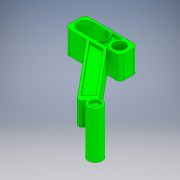
# Autodesk Inventor part: finger_4_6mm
Saved by Autodesk Inventor 2018 (Build 220112000, 112)
## iProperties
Created: 2019-01-24
Part Number: finger_4_6mm
Material: 一般
Document SubType Name: Modeling
Designer: lowyu
Density: 1 g/cm^3
Appearance: 既定
Author: lowyu
## iProperties of the stored document finger_4_6mm_3D プリント.ipt
Created: 2019-01-24
Part Number: finger_4_6mm_3D プリント
Material: 一般
Document SubType Name: Modeling
Designer: lowyu
Density: 1 g/cm^3
Appearance: 既定
Author: lowyu
Autodesk Inventor part; units mm, degrees
ref_plane "YZ Plane" through (0, 0, 0) normal (1, 0, 0) x (0, 1, 0)
ref_plane "XZ Plane" through (0, 0, 0) normal (0, 1, 0) x (-1, 0, 0)
ref_plane "XY Plane" through (0, 0, 0) normal (0, 0, 1) x (1, 0, 0)
sketch "スケッチ1" plane through (0, 0, 0) normal (0, 0, 1) x (1, 0, 0)
  line L0 (18.4549, -7.695) -> (14.2688, -7.695)
  arc A0 (18.4549, -7.695) -> (20.0703, -6.0796) centre (18.4549, -6.0796) ccw
  line L1 (20.0703, -2.0624) -> (20.0703, -6.0796)
  line L2 (18.0495, -0.0417) -> (-1.0589, -0.0417)
  arc A1 (-1.0589, -0.0417) -> (-2.9016, -1.8843) centre (-1.0589, -1.8843) ccw
  line L3 (-2.9016, -1.8843) -> (-2.9016, -6.5999)
  arc A2 (-2.9016, -6.5999) -> (-0.7003, -8.8011) centre (-0.7003, -6.5999) ccw
  arc A3 (26.8872, -33.0759) -> (27.9503, -33.1763) centre (27.7277, -29.8571) ccw
  line L4 (29.6628, -31.7291) -> (27.9503, -33.1763)
  arc A4 (29.6628, -31.7291) -> (31.463, -28.2522) centre (32.5816, -31.0359) ccw
  line L5 (31.463, -28.2522) -> (14.2688, -7.695)
  circle A5 centre (16.1123, -4.0657) radius 2.5
  line L6 (7.6373, -0.9827) -> (1.1644, -0.9827)
  arc A6 (7.6373, -7.2327) -> (7.6373, -0.9827) centre (7.6373, -4.1077) ccw
  arc A7 (1.1644, -0.9827) -> (1.1644, -7.2327) centre (1.1644, -4.1077) ccw
  line L7 (26.8872, -33.0759) -> (6.5837, -8.8011)
  line L8 (-0.7003, -8.8011) -> (6.5837, -8.8011)
  arc A8 (20.0703, -2.0624) -> (18.0495, -0.0417) centre (18.0495, -2.0624) ccw
  line L9 (1.1644, -7.2327) -> (7.6373, -7.2327)
  line L10 (13.6123, -4.0657) -> (13.6123, 1.3375)
  line L11 (10.7623, -4.0657) -> (10.7623, 0.9924)
  point P0 (0, 0)
  point P1 (0, 0)
  point P2 (0, 0)
  dimension "d0" = 5
  dimension "d1" = 3.125
  dimension "d2" = 4.8539
  dimension "d3" = 4.066
  dimension "d4" = 4.066
  dimension "d5" = 90
  dimension "d6" = 90
  dimension "d7" = 3.125
  dimension "d8" = 3.9579
  dimension "d9" = 22.9718
  dimension "d10" = 3
  dimension "d11" = 2.85
  constraints: 24 end point, 16 point on circle, 11 tangent, 8 centre point, 4 parallel, 2 horizontal, 2 perpendicular, 1 coincident, 1 horizontal alignment, 1 vertical, 2 other
  measures "d1" radius of A6
  measures "d2" horizontal distance of A4.centre A3.centre
  measures "d3" distance from line of L2 A7.centre
  measures "d4" distance from line of L3 A7.centre
  measures "d7" radius of A7
  measures "d8" distance from line of L1 point (16.112, -4.066)
  measures "d9" distance between parallel lines of L1 L3
  measures "d10" radius of A4
  measures "d11" distance between parallel lines of L10 L11
extrude "押し出し1" add sketch "スケッチ1" along normal blind 10
sketch "スケッチ2" plane through (0, 0, 0) normal (0, 0, -1) x (-1, 0, 0)
  arc A0 (-31.463, -28.2522) -> (-29.6628, -31.7291) centre (-32.5816, -31.0359) ccw projected
  circle A1 centre (-32.5816, -31.0359) radius 3
  point P0 (0, 0)
  constraints: 1 centre point, 1 coincident, 1 concentric
extrude "押し出し2" add sketch "スケッチ2" along normal blind 10
sketch "スケッチ3" plane through (0, 0, 10) normal (0, 0, 1) x (1, 0, 0)
  line L0 (6.5837, -8.8011) -> (26.8872, -33.0759) projected
  line L1 (31.463, -28.2522) -> (14.2688, -7.695) projected
  line L2 (6.5837, -8.8011) -> (15.194, -8.8011)
  line L3 (26.8872, -33.0759) -> (31.463, -28.2522)
  line L4 (31.463, -28.2522) -> (15.194, -8.8011)
  line L5 (26.8872, -33.0759) -> (6.5837, -8.8011)
  line L6 (25.9184, -31.9176) -> (30.4942, -27.0939)
  line L7 (26.6112, -31.1873) -> (7.8873, -8.8011)
  line L8 (29.8014, -27.8243) -> (13.8903, -8.8011)
  point P0 (0, 0)
  dimension "d16" = 1.5
  dimension "d17" = 1
  dimension "d18" = 1
  constraints: 14 end point, 7 point on line, 3 parallel, 1 collinear, 1 horizontal
  measures "d16" distance between parallel lines of L3 L6
  measures "d17" distance between parallel lines of L0 L7
  measures "d18" distance between parallel lines of L1 L8
extrude "押し出し3" cut sketch "スケッチ3" against normal blind 1 contours L2 L8 L6 L7
sketch "スケッチ4" plane through (0, 0, 10) normal (0, 0, 1) x (1, 0, 0)
  arc A0 (7.6373, -7.2327) -> (7.6373, -0.9827) centre (7.6373, -4.1077) ccw projected
  circle A1 centre (16.1123, -4.0657) radius 2.5 projected
  line L0 (18.0495, -0.0417) -> (-1.0589, -0.0417) projected
  line L1 (14.2688, -7.695) -> (18.4549, -7.695) projected
  line L2 (7.8873, -8.8011) -> (13.8903, -8.8011) projected
  line L3 (13.8903, -8.8011) -> (29.8014, -27.8243) projected
  line L4 (29.8014, -27.8243) -> (26.6112, -31.1873) projected
  line L5 (26.6112, -31.1873) -> (7.8873, -8.8011) projected
  line L6 (7.8873, -8.8011) -> (13.8903, -8.8011) projected
  arc A2 (7.6373, -7.2327) -> (7.6373, -0.9827) centre (7.6373, -4.1077) ccw projected
  line L7 (7.6373, -7.2327) -> (1.1644, -7.2327) projected
  arc A3 (1.1644, -0.9827) -> (1.1644, -7.2327) centre (1.1644, -4.1077) ccw projected
  line L8 (1.1644, -0.9827) -> (7.6373, -0.9827) projected
  circle A4 centre (16.1123, -4.0657) radius 2.5 projected
  line L9 (14.2688, -7.695) -> (18.4549, -7.695) projected
  arc A5 (18.4549, -7.695) -> (20.0703, -6.0796) centre (18.4549, -6.0796) ccw projected
  line L10 (20.0703, -6.0796) -> (20.0703, -2.0624) projected
  arc A6 (20.0703, -2.0624) -> (18.0495, -0.0417) centre (18.0495, -2.0624) ccw projected
  line L11 (18.0495, -0.0417) -> (-1.0589, -0.0417) projected
  arc A7 (-1.0589, -0.0417) -> (-2.9016, -1.8843) centre (-1.0589, -1.8843) ccw projected
  line L12 (-2.9016, -1.8843) -> (-2.9016, -6.5999) projected
  arc A8 (-2.9016, -6.5999) -> (-0.7003, -8.8011) centre (-0.7003, -6.5999) ccw projected
  line L13 (-0.7003, -8.8011) -> (6.5837, -8.8011) projected
  line L14 (6.5837, -8.8011) -> (26.8872, -33.0759) projected
  arc A9 (26.8872, -33.0759) -> (27.9503, -33.1763) centre (27.7277, -29.8571) ccw projected
  line L15 (27.9503, -33.1763) -> (29.6628, -31.7291) projected
  arc A10 (29.6628, -31.7291) -> (31.463, -28.2522) centre (32.5816, -31.0359) ccw projected
  line L16 (31.463, -28.2522) -> (14.2688, -7.695) projected
  arc A11 (9.5454, -7.2327) -> (9.5355, -0.9767) centre (7.6373, -4.1077) ccw
  arc A12 (14.3143, -0.9767) -> (14.4552, -7.2327) centre (16.1123, -4.0657) ccw
  line L17 (9.5454, -7.2327) -> (14.4552, -7.2327)
  line L18 (9.5355, -0.9767) -> (14.3143, -0.9767)
  point P0 (0, 0)
  constraints: 5 point on circle, 4 end point, 2 centre point, 2 coincident, 2 horizontal
extrude "押し出し4" cut sketch "スケッチ4" against normal blind 1 contours A11 L18 A12 L17
sketch "スケッチ5" plane through (0, 0, 10) normal (0, 0, 1) x (1, 0, 0)
  arc A0 (29.6628, -31.7291) -> (31.463, -28.2522) centre (32.5816, -31.0359) ccw projected
  circle A1 centre (32.5816, -31.0359) radius 2
  circle A2 centre (32.5816, -31.0359) radius 3
  point P0 (0, 0)
  dimension "d23" = 1
  dimension "d24" = 1
  constraints: 2 centre point, 2 coincident
  measures "d23" radial gap between concentric circles of A1 A0
  measures "d24" radial gap between concentric circles of A1 A2
extrude "押し出し5" cut sketch "スケッチ5" against normal blind 1 contours A1
equation "\"d4\" = d3"
equation "\"d7\" = d1"
